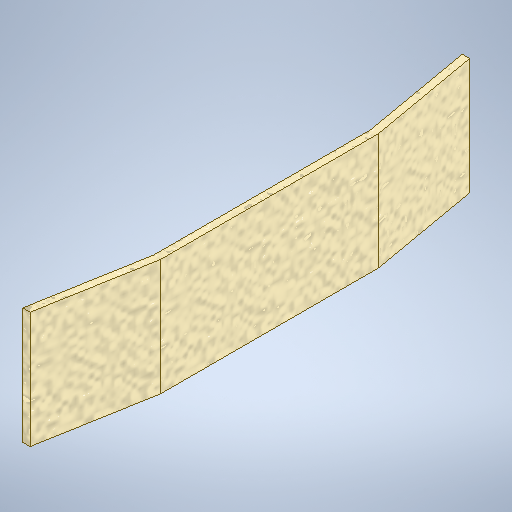
# Autodesk Inventor part: guia
Saved by Autodesk Inventor 2025.2 (Build 292293000, 293)
## iProperties
Created: 2025-11-13
Part Number: guia
Material: Genérico
Document SubType Name: Modeling
Designer: Dax
Density: 1 g/cm^3
Appearance: Fino - Crema
Author: Dax
Autodesk Inventor part; units mm, degrees
ref_plane "YZ Plane" through (0, 0, 0) normal (1, 0, 0) x (0, 1, 0)
ref_plane "XZ Plane" through (0, 0, 0) normal (0, 1, 0) x (-1, 0, 0)
ref_plane "XY Plane" through (0, 0, 0) normal (0, 0, 1) x (1, 0, 0)
sketch "Boceto1" plane through (0, 0, 0) normal (0, 1, 0) x (-1, 0, 0)
  line L0 (-287, -225) -> (-287, -75)
  line L1 (-287, -225) -> (-287, -175)
  line L2 (-287, -175) -> (-287, -225)
  line L3 (-287, -225) -> (-273.5759, -301.1318)
  line L4 (-287, -225) -> (-287, -75)
  line L5 (-287, -75) -> (-273.5759, 1.1318)
  line L6 (-282, -225) -> (-282, -75)
  line L7 (-282.076, -224.1318) -> (-268.4988, -301.1318)
  line L8 (-282.076, -75.8682) -> (-268.4988, 1.1318)
  line L9 (-268.4988, 1.1318) -> (-273.5759, 1.1318)
  line L10 (-268.4988, -301.1318) -> (-273.5759, -301.1318)
  point P0 (0, 0)
  point P1 (-282, -224.5626)
  point P2 (-282, -75.4374)
  dimension "d5" = 170
  dimension "d7" = 170
  dimension "d9" = 5
  dimension "d10" = 5
  dimension "d11" = 5
  constraints: 22 end point, 4 parallel, 1 horizontal, 1 point on line
  measures "d5" angle of L3 L2
  measures "d7" angle of L4 L5
  measures "d9" distance between parallel lines of L0 L6
  measures "d10" distance between parallel lines of L3 L7
  measures "d11" distance between parallel lines of L5 L8
extrude "Extrusión1" add sketch "Boceto1" along normal blind 80
